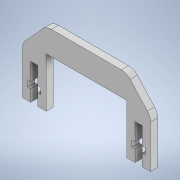
# Autodesk Inventor part: крепление_аккума
Saved by Autodesk Inventor 2021.1 (Build 251245010, 245A)
## iProperties
Created: 2023-02-15
Part Number: крепление_аккума
Material: Типовые
Document SubType Name: Modeling
Designer: zmoze
Density: 1 g/cm^3
Appearance: По умолчанию
Author: zmoze
Autodesk Inventor part; units mm, degrees
ref_plane "YZ Plane" through (0, 0, 0) normal (1, 0, 0) x (0, 1, 0)
ref_plane "XZ Plane" through (0, 0, 0) normal (0, 1, 0) x (-1, 0, 0)
ref_plane "XY Plane" through (0, 0, 0) normal (0, 0, 1) x (1, 0, 0)
sketch "Эскиз1" plane through (0, 0, 0) normal (0, 0, 1) x (1, 0, 0)
  line L0 (-17, 0) -> (-27, 0)
  line L1 (-27, 0) -> (-27, 20)
  line L2 (-27, 20) -> (-17, 31)
  line L3 (-17, 31) -> (17, 31)
  line L4 (17, 31) -> (27, 20)
  line L5 (27, 20) -> (27, 0)
  line L6 (27, 0) -> (17, 0)
  line L7 (17, 0) -> (17, 21)
  line L8 (17, 21) -> (-17, 21)
  line L9 (-17, 21) -> (-17, 0)
  line L10 (0, 0) -> (0, 29.9974) construction
  line L11 (-23.5, 0) -> (-23.5, 5)
  line L12 (-23.5, 5) -> (-24.8, 5)
  line L13 (-24.8, 5) -> (-24.8, 7.6)
  line L14 (-24.8, 7.6) -> (-23.5, 7.6)
  line L15 (-23.5, 7.6) -> (-23.5, 15)
  line L16 (-23.5, 15) -> (-20.5, 15)
  line L17 (-20.5, 15) -> (-20.5, 7.6)
  line L18 (-20.5, 7.6) -> (-19.2, 7.6)
  line L19 (-19.2, 7.6) -> (-19.2, 5)
  line L20 (-19.2, 5) -> (-20.5, 5)
  line L21 (-20.5, 5) -> (-20.5, 0)
  line L22 (-23.5, 0) -> (-20.5, 0)
  line L23 (20.5, 0) -> (20.5, 5)
  line L24 (20.5, 5) -> (19.2, 5)
  line L25 (19.2, 5) -> (19.2, 7.6)
  line L26 (19.2, 7.6) -> (20.5, 7.6)
  line L27 (20.5, 7.6) -> (20.5, 15)
  line L28 (20.5, 15) -> (23.5, 15)
  line L29 (23.5, 15) -> (23.5, 7.6)
  line L30 (23.5, 7.6) -> (24.8, 7.6)
  line L31 (24.8, 7.6) -> (24.8, 5)
  line L32 (24.8, 5) -> (23.5, 5)
  line L33 (23.5, 5) -> (23.5, 0)
  line L34 (-22, 0) -> (-22, 10.9086) construction
  line L35 (22, 0) -> (22, 13.2946) construction
  point P0 (0, 21)
  point P1 (0, 31)
  point P2 (-22, 15)
  point P3 (22, 15)
  point P4 (-20.5, 0)
  dimension "d0" = 34
  dimension "d1" = 21
  dimension "d3" = 20
  dimension "d4" = 34
  dimension "d5" = 10
  dimension "d6" = 10
  dimension "d10" = 3
  dimension "d11" = 2.6
  dimension "d12" = 5
  dimension "d13" = 15
  dimension "d14" = 5.6
  constraints: 72 end point, 20 point on line, 12 perpendicular, 8 vertical, 7 collinear, 6 equal length, 6 midpoint, 4 parallel, 2 horizontal
  measures "d0" distance of L7.end L8.end
  measures "d1" distance of L6.end L7.end
  measures "d3" distance of L4.end L5.end
  measures "d4" distance of L2.end L3.end
  measures "d5" distance between parallel lines of L8 L3
  measures "d6" distance between parallel lines of L9 L1
  measures "d10" distance of L15.end L16.end
  measures "d11" distance of L18.end L19.end
  measures "d12" distance between parallel lines of L0 L20
  measures "d13" distance between parallel lines of L0 L16
  measures "d14" distance between parallel lines of L19 L13
extrude "Выдавливание1" add sketch "Эскиз1" along normal blind 3 contours L0 L21 L20 L19 L18 L17 L16 L15 L14 L13 L12 L11 L1 L2 L3 L4 L5 L6 L33 L32 L31 L30 L29 L28 L27 L26 L25 L24 L23 L7 L8 L9
fillet "Сопряжение1" radius 5 4 edges at (17, 31, 1.5) (27, 20, 1.5) (-17, 31, 1.5) (-27, 20, 1.5)
